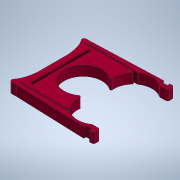
# Autodesk Inventor part: fast_battery3_2
Saved by Autodesk Inventor 2020 (Build 240168000, 168)
## iProperties
Created: 2022-07-19
Part Number: fast_battery3_2
Material: Типовые
Document SubType Name: Modeling
Designer: akapu
Density: 1 g/cm^3
Appearance: По умолчанию
Author: akapu
Autodesk Inventor part; units mm, degrees
ref_plane "YZ Plane" through (0, 0, 0) normal (1, 0, 0) x (0, 1, 0)
ref_plane "XZ Plane" through (0, 0, 0) normal (0, 1, 0) x (-1, 0, 0)
ref_plane "XY Plane" through (0, 0, 0) normal (0, 0, 1) x (1, 0, 0)
sketch "Эскиз6" plane through (0, 0, 0) normal (0, 1, 0) x (-1, 0, 0)
  line L0 (0, 0) -> (-42.988, 0)
  line L1 (-42.988, 0) -> (-42.988, -36.6)
  line L2 (-42.988, -36.6) -> (0, -36.6)
  line L3 (0, -36.6) -> (0, 0)
  line L4 (-42.988, -36.6) -> (-33.688, -36.6)
  circle A0 centre (-33.688, -9.3) radius 9.3
  circle A1 centre (-33.688, -27.3) radius 9.3
  circle A2 centre (-18.0995, -18.3) radius 9.3
  line L5 (-6.4995, -34.6) -> (-6.4995, -2)
  line L6 (-6.4995, 0) -> (-6.4995, -4)
  line L7 (-6.4995, -4) -> (-7.5995, -4)
  line L8 (-6.4995, -34.6) -> (-6.4995, -32.6)
  line L9 (-6.4995, -32.6) -> (-7.5995, -32.6)
  line L10 (-6.4995, -34.6) -> (-6.4995, -36.6)
  line L11 (-6.4995, 0) -> (-3.4995, 0)
  line L12 (-3.4995, 0) -> (-3.4995, -36.6)
  line L13 (-3.4995, -36.6) -> (-6.4995, -36.6)
  line L14 (-6.4995, -36.6) -> (-6.4995, 0)
  line L15 (-7.5995, -4) -> (-7.5995, -32.6)
  line L16 (0, 0) -> (0, -1)
  line L17 (0, -36.6) -> (0, -35.6)
  line L18 (0, -1) -> (-3.4995, -18)
  line L19 (-3.4995, -18) -> (0, -35.6)
  line L20 (-1.7498, -26.8) -> (-3.4995, -34.6)
  line L21 (-1.7498, -9.5) -> (-3.4995, -2)
  spline S0 degree 2 poles (0, -1) (-4.3156, -5.2461) (-3.5613, -18.3) knots 0 0 0 1 1 1
  spline S1 degree 2 poles (0, -35.6) (-4.3216, -31.1884) (-3.4995, -18) knots 0 0 0 1 1 1
  point P0 (-33.688, 0)
  point P1 (-24.7222, -11.7708)
  point P2 (-24.7222, -24.8292)
  point P3 (-2.6247, -5.75)
  point P4 (-2.6247, -30.7)
  point P5 (-3.4995, -25.5342)
  point P6 (-3.4995, -10.5622)
  dimension "d38" = 42.988
  dimension "d39" = 36.6
  dimension "d44" = 18.6
  dimension "d48" = 32.6
  dimension "d51" = 3
  dimension "d52" = 1
  dimension "d53" = 1
  constraints: 44 end point, 12 point on line, 5 parallel, 4 midpoint, 4 perpendicular, 2 centre point, 2 horizontal, 9 other
  measures "d38" distance of L2.end L1.end
  measures "d39" distance of L1.end L0.end
  measures "d44" diameter of A2
  measures "d48" distance of L5.start L5.end
  measures "d51" distance of L12.end L13.end
  measures "d52" distance of L0.start L16.end
  measures "d53" distance of L2.end L17.end
extrude "Выдавливание5" add sketch "Эскиз6" along normal blind 5 contours L3 S0 L21 L12 L0 | L12 S1 L2 L10 L5 L6 L0 | L6 L5 L7 L15 L9 L10 L2 A1 A2 A0 L0 | L21 S0 L12 | L3 L2 L12 L20 S1 | L20 L12 S1 | L12 S1
fillet "Сопряжение1" radius 0.5 4 edges at (24.7222, 2.5, -24.8292) (33.688, 2.5, -36.6) (24.7222, 2.5, -11.7708) (33.688, 2.5, 0)
sketch "Эскиз7" plane through (0, 5, 0) normal (0, 1, 0) x (1, 0, 0)
  arc A0 (24.4513, 10.3832) -> (29.5953, 0.949) centre (33.688, 9.3) ccw projected
  circle A1 centre (33.688, 9.3) radius 9.3
  line L0 (42.988, 0) -> (42.988, 36.6)
  line L1 (29.3752, 36.6) -> (0, 36.6) projected
  line L2 (42.988, 36.6) -> (0, 36.6)
  line L3 (0, 0) -> (29.3752, 0) projected
  line L4 (0, 36.6) -> (0, 0)
  line L5 (0, 0) -> (42.988, 0)
  arc A2 (29.5953, 35.651) -> (24.4513, 26.2168) centre (33.688, 27.3) ccw projected
  circle A3 centre (33.688, 27.3) radius 9.3
  arc A4 (23.656, 25.7576) -> (23.656, 10.8424) centre (18.0995, 18.3) ccw projected
  circle A5 centre (18.0995, 18.3) radius 9.3
  line L6 (18.0995, 9) -> (18.0995, 0)
  line L7 (18.0995, 4.5) -> (25.7224, 4.5)
  line L8 (18.0995, 27.6) -> (18.0995, 36.6)
  line L9 (18.0995, 32.1) -> (25.7224, 32.1)
  circle A6 centre (21.911, 4.5) radius 1.6
  circle A7 centre (21.911, 32.1) radius 1.6
  line L10 (3.4995, 25.5342) -> (3.4995, 10.5622) projected
  line L11 (3.4995, 3.4558) -> (3.4995, 0)
  line L12 (3.4995, 1.7279) -> (42.988, 1.7279)
  line L13 (42.988, 1.7279) -> (42.988, -1.4721)
  line L14 (42.988, -1.4721) -> (3.4995, 0)
  line L15 (42.988, -1.4721) -> (41.489, -1.4162)
  line L16 (3.4995, 1.7279) -> (3.4995, 2.1279)
  line L17 (3.4995, 2.1279) -> (27.7676, 2.1279)
  line L18 (42.988, -1.4721) -> (42.988, -0.4721)
  line L19 (3.4995, 0) -> (3.4995, 1)
  line L20 (3.4995, 33.1442) -> (3.4995, 36.6)
  line L21 (3.4995, 36.6) -> (3.4995, 34.872)
  line L22 (3.4995, 34.872) -> (28.2885, 34.872)
  point P0 (39.0874, 1.7279)
  point P1 (29.5953, 0.949)
  point P2 (28.2886, 1.7279)
  dimension "d58" = 36.6
  dimension "d60" = 3.2
  dimension "d61" = 3.2
  dimension "d62" = 3.2
  dimension "d63" = 1.5
  dimension "d64" = 0.4
  dimension "d71" = 1
  dimension "d72" = 1
  dimension "d73" = 1.728
  constraints: 40 end point, 14 point on line, 7 perpendicular, 6 point on circle, 5 centre point, 5 midpoint, 3 coincident, 3 vertical, 1 parallel
  measures "d58" distance of L0.start L0.end
  measures "d60" diameter of A6
  measures "d61" diameter of A7
  measures "d62" distance of L12.end L13.end
  measures "d63" distance of L13.end L15.end
  measures "d64" distance of L12.start L16.end
  measures "d71" distance of L13.end L18.end
  measures "d72" distance of L11.end L19.end
  measures "d73" distance of L20.end L21.end
extrude "Выдавливание6" add sketch "Эскиз7" against normal blind 5 contours A0 A1 L5 L3 L6 L12 | L6 L3 L11 L12 | L12 L0 L5 A1 | L5 L13 L14 L3
sketch "Эскиз8" plane through (0, 5, 0) normal (0, 1, 0) x (1, 0, 0)
  line L0 (3.4995, 3.4558) -> (3.4995, 2.1278)
  line L1 (3.4995, 2.1278) -> (27.7678, 2.1278)
  arc A0 (24.4513, 10.3832) -> (39.0874, 1.7279) centre (33.688, 9.3) ccw projected
  line L2 (3.4995, 2.1278) -> (3.4995, 1.7278)
  line L3 (3.4995, 1.7278) -> (28.2888, 1.7278)
  line L4 (28.2888, 1.7278) -> (29.5707, 1.7278)
  line L5 (29.5707, 1.7278) -> (28.9297, 2.3739)
  line L6 (28.9297, 2.3739) -> (27.7678, 2.1278)
  point P0 (0, 0)
  dimension "d67" = 1.328
  dimension "d68" = 0.4
  constraints: 14 end point, 2 perpendicular, 2 point on circle, 2 point on line, 1 vertical
  measures "d67" distance of L0.start L0.end
  measures "d68" distance of L0.end L2.end
extrude "Выдавливание7" cut sketch "Эскиз8" against normal blind 5
sketch "Эскиз9" plane through (0, 5, 0) normal (0, 1, 0) x (1, 0, 0)
  line L0 (27.7678, 2.1278) -> (3.4995, 2.1278) projected
  line L1 (29.3752, 36.6) -> (0, 36.6) projected
  line L2 (3.4995, 25.5342) -> (3.4995, 33.9682)
  arc A0 (29.5953, 35.651) -> (24.4513, 26.2168) centre (33.688, 27.3) ccw projected
  circle A1 centre (33.688, 27.3) radius 9.3
  line L3 (3.4995, 36.6) -> (3.4995, 34.872)
  line L4 (3.4995, 34.872) -> (28.2885, 34.872)
  arc A2 (29.5953, 35.651) -> (24.4513, 26.2168) centre (33.688, 27.3) ccw projected
  line L5 (3.4995, 34.872) -> (3.4995, 34.472)
  line L6 (3.4995, 34.472) -> (28.0497, 34.472)
  line L7 (28.0497, 34.472) -> (28.2885, 34.872)
  point P0 (0, 0)
  point P1 (27.7675, 34.472)
  dimension "d74" = 8.434
  dimension "d78" = 1.728
  dimension "d79" = 0.4
  constraints: 12 end point, 2 perpendicular, 2 point on line, 1 centre point, 1 coincident, 1 concentric, 1 point on circle, 1 vertical
  measures "d74" distance of L2.start L2.end
  measures "d78" distance of L3.start L3.end
  measures "d79" distance of L3.end L5.end
extrude "Выдавливание8" cut sketch "Эскиз9" against normal blind 5 contours A0 L6 L5 L4
sketch "Эскиз10" plane through (0, 5, 0) normal (0, 1, 0) x (1, 0, 0)
  line L0 (29.3752, 36.6) -> (0, 36.6) projected
  arc A0 (27.7675, 34.472) -> (24.4513, 26.2168) centre (33.688, 27.3) ccw projected
  circle A1 centre (33.688, 27.3) radius 9.3
  arc A2 (24.4513, 10.3832) -> (27.7678, 2.1278) centre (33.688, 9.3) ccw projected
  circle A3 centre (33.688, 9.3) radius 9.3
  line L1 (39.0874, 1.7279) -> (42.988, 1.7279) projected
  line L2 (3.4995, 2.1278) -> (3.4995, 34.472)
  line L3 (25.7638, 2.1278) -> (25.7638, 34.472)
  line L4 (27.7675, 34.472) -> (3.4995, 34.472) projected
  line L5 (42.988, 9.3) -> (42.988, 27.3)
  line L6 (42.988, 9.3) -> (42.988, 1.7279)
  line L7 (42.988, 27.3) -> (42.988, 34.872)
  line L8 (3.4995, 34.872) -> (3.4995, 34.472) projected
  line L9 (42.988, 34.872) -> (3.4995, 34.872)
  line L10 (42.988, 34.872) -> (42.988, 38.072)
  line L11 (42.988, 38.072) -> (3.4995, 36.6)
  line L12 (3.4995, 34.872) -> (3.4995, 36.6)
  line L13 (42.988, 38.072) -> (40.9894, 37.9975)
  line L14 (40.9894, 37.9975) -> (41.0341, 36.7983)
  line L15 (41.0341, 36.7983) -> (38.0362, 36.6866)
  line L16 (38.0362, 36.6866) -> (37.9915, 37.8857)
  point P0 (0, 0)
  point P1 (28.2885, 34.872)
  point P2 (39.0875, 34.872)
  dimension "d83" = 32.3442
  dimension "d84" = 32.3442
  dimension "d86" = 7.5721
  dimension "d88" = 7.572
  dimension "d89" = 3.2
  dimension "d90" = 2
  dimension "d91" = 1.2
  dimension "d92" = 3
  constraints: 26 end point, 5 point on line, 4 perpendicular, 4 vertical, 2 coincident, 2 tangent, 1 centre point, 1 point on circle, 3 other
  measures "d83" distance of L3.start L3.end
  measures "d84" distance of L2.start L2.end
  measures "d86" distance of L5.start L1.end
  measures "d88" distance of L5.end L7.end
  measures "d89" distance of L7.end L10.end
  measures "d90" distance of L10.end L13.end
  measures "d91" distance of L13.end L14.end
  measures "d92" distance of L14.end L15.end
extrude "Выдавливание9" add sketch "Эскиз10" against normal blind 5 contours L9 L12 L11 L16 L15 L14 L10 A1
sketch "Эскиз11" plane through (0, 5, 0) normal (0, 1, 0) x (1, 0, 0)
  line L0 (42.988, 1.7279) -> (42.988, -1.4721) projected
  line L1 (42.988, -1.4721) -> (40.9894, -1.3976)
  line L2 (42.988, -1.4721) -> (3.4995, 0) projected
  line L3 (40.9894, -1.3976) -> (41.0341, -0.1984)
  line L4 (41.0341, -0.1984) -> (38.0362, -0.0867)
  line L5 (38.0362, -0.0867) -> (37.9915, -1.2858)
  line L6 (37.9915, -1.2858) -> (40.9894, -1.3976)
  point P0 (0, 0)
  dimension "d95" = 2
  dimension "d96" = 1.2
  dimension "d97" = 3
  constraints: 10 end point, 4 perpendicular, 2 point on line
  measures "d95" distance of L0.end L1.end
  measures "d96" distance of L1.end L3.end
  measures "d97" distance of L3.end L4.end
extrude "Выдавливание10" cut sketch "Эскиз11" against normal blind 5
fillet "Сопряжение3" radius 0.5 6 edges at (27.7678, 2.5, -2.1278) (28.2888, 2.5, -1.7278) (27.7675, 2.5, -34.472) (28.2885, 2.5, -34.872) (39.0875, 2.5, -34.872) (39.0874, 2.5, -1.7279)
fillet "Сопряжение4" radius 1 8 edges at (42.988, 2.5, 1.4721) (42.988, 2.5, -1.7279) (42.988, 2.5, -34.872) (42.988, 2.5, -38.072) (0, 2.5, -1) (0, 2.5, 0) (0, 2.5, -35.6) (0, 2.5, -36.6)
